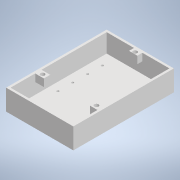
# Autodesk Inventor part: корпус
Saved by Autodesk Inventor 2022 (Build 260153000, 153)
## iProperties
Created: 2022-10-20
Part Number: корпус
Material: Типовые
Document SubType Name: Modeling
Designer: Robo0
Density: 1 g/cm^3
Appearance: По умолчанию
Author: Robo0
Autodesk Inventor part; units mm, degrees
ref_plane "YZ Plane" through (0, 0, 0) normal (1, 0, 0) x (0, 1, 0)
ref_plane "XZ Plane" through (0, 0, 0) normal (0, 1, 0) x (-1, 0, 0)
ref_plane "XY Plane" through (0, 0, 0) normal (0, 0, 1) x (1, 0, 0)
sketch "Эскиз1" plane through (0, 0, 0) normal (0, 1, 0) x (-1, 0, 0)
  line L0 (0, 0) -> (200, 0)
  line L1 (200, 0) -> (200, 200)
  line L2 (200, 200) -> (0, 200)
  line L3 (0, 200) -> (0, 0)
  dimension "d0" = 200
  dimension "d1" = 200
  constraints: 8 end point, 2 parallel, 1 horizontal, 1 perpendicular
  measures "d0" distance of L2.end L1.end
  measures "d1" distance of L1.end L0.end
extrude "Выдавливание1" add sketch "Эскиз1" along normal blind 3
sketch "Эскиз2" plane through (0, 3, 0) normal (0, 1, 0) x (1, 0, 0)
  line L0 (-200, 0) -> (-200, -200) projected
  line L1 (-200, -200) -> (0, -200) projected
  line L2 (0, -200) -> (0, 0) projected
  line L3 (0, 0) -> (-200, 0) projected
  line L4 (0, -200) -> (0, 0) projected
  line L5 (0, 0) -> (-90.778, 0)
  line L6 (-90.778, 0) -> (-90.778, -135.834)
  line L7 (-90.778, -135.834) -> (0, -135.834)
  line L8 (0, -135.834) -> (0, 0)
  constraints: 8 end point, 2 parallel, 1 horizontal, 1 perpendicular
extrude "Выдавливание2" cut sketch "Эскиз2" against normal blind 3 contours L3 L6 L7 L2 L1 L0
sketch "Эскиз3" plane through (0, 3, 0) normal (0, 1, 0) x (1, 0, 0)
  line L0 (-90.778, 0) -> (-90.778, -135.834) projected
  line L1 (-90.778, -135.834) -> (0, -135.834) projected
  line L2 (0, -135.834) -> (0, 0) projected
  line L3 (0, 0) -> (-90.778, 0) projected
  line L4 (-87.778, -132.834) -> (-3, -132.834)
  line L5 (-3, -132.834) -> (-3, -3)
  line L6 (-3, -3) -> (-87.778, -3)
  line L7 (-87.778, -3) -> (-87.778, -132.834)
  dimension "d6" = 3
  dimension "d7" = 3
  dimension "d8" = 3
  dimension "d9" = 3
  constraints: 8 end point, 2 parallel, 1 horizontal, 1 perpendicular
  measures "d6" distance between parallel lines of L0 L7
  measures "d7" distance between parallel lines of L6 L3
  measures "d8" distance between parallel lines of L2 L5
  measures "d9" distance between parallel lines of L1 L4
extrude "Выдавливание3" add sketch "Эскиз3" along normal blind 25
sketch "Эскиз4" plane through (0, 28, 0) normal (0, 1, 0) x (1, 0, 0)
  line L0 (-87.778, -3) -> (-3, -3) projected
  line L1 (-87.778, -132.834) -> (-87.778, -3) projected
  line L2 (-3, -3) -> (-3, -132.834) projected
  circle A0 centre (-81.778, -95.6228) radius 2.75
  circle A1 centre (-9, -95.6228) radius 2.75
  circle A2 centre (-45.389, -7) radius 2.75
  line L3 (-87.778, -99.5857) -> (-76.0264, -99.5857)
  line L4 (-76.0264, -99.5857) -> (-76.0264, -91)
  line L5 (-76.0264, -91) -> (-87.778, -91)
  line L6 (-87.778, -91) -> (-87.778, -99.5857)
  line L7 (-50.872, -3) -> (-39.6049, -3)
  line L8 (-39.6049, -3) -> (-39.6049, -9.75)
  line L9 (-39.6049, -9.75) -> (-50.872, -9.75)
  line L10 (-50.872, -9.75) -> (-50.872, -3)
  line L11 (-3, -91) -> (-13.2714, -91)
  line L12 (-13.2714, -91) -> (-13.2714, -100.2408)
  line L13 (-13.2714, -100.2408) -> (-3, -100.2408)
  line L14 (-3, -100.2408) -> (-3, -91)
  line L15 (-36, -90) -> (-62, -90) projected
  point P0 (0, 0)
  point P1 (-45.389, -9.75)
  point P2 (-3, -100.2408)
  dimension "d12" = 5.5
  dimension "d13" = 6
  dimension "d14" = 5.5
  dimension "d15" = 6
  dimension "d16" = 5.5
  dimension "d17" = 4
  dimension "d18" = 1
  dimension "d19" = 4.6227
  constraints: 24 end point, 6 parallel, 4 point on line, 3 centre point, 3 horizontal, 3 perpendicular
  measures "d12" diameter of A0
  measures "d13" distance from line of A0.centre L1
  measures "d14" diameter of A1
  measures "d15" distance from line of A1.centre L2
  measures "d16" diameter of A2
  measures "d17" distance from line of A2.centre L0
  measures "d18" distance between parallel lines of L5 L15
  measures "d19" distance from line of L5 A0.centre
extrude "Выдавливание4" add sketch "Эскиз4" against normal blind 10
sketch "Эскиз5" plane through (-90.778, 0, 0) normal (-1, 0, 0) x (0, 0, 1)
  point P0 (0, 0)
sketch "Эскиз6" plane through (-90.778, 0, 0) normal (-1, 0, 0) x (0, 0, 1)
  line L0 (123, 6.5) -> (123, 0.5) projected
  line L1 (129, 6.5) -> (123, 6.5) projected
  line L2 (129, 0.5) -> (129, 6.5) projected
  line L3 (129.6397, 6.975) -> (122.4748, 6.975)
  line L4 (122.4748, 6.975) -> (122.4748, 0.5)
  line L5 (122.4748, 0.5) -> (129.6397, 0.5)
  line L6 (129.6397, 0.5) -> (129.6397, 6.975)
  point P0 (0, 0)
  constraints: 8 end point, 2 parallel, 1 horizontal, 1 perpendicular
extrude "Выдавливание5" cut sketch "Эскиз6" against normal blind 10
sketch "Эскиз7" plane through (0, 0, 0) normal (0, -1, 0) x (1, 0, 0)
  spline S0 degree 3 poles (-76.75, 18.5) (-76.7941, 18.5) (-76.8383, 18.5019) (-76.8822, 18.5058) (-76.939, 18.5109) (-76.9955, 18.5191) (-77.0514, 18.5306) (-77.1245, 18.5456) (-77.1965, 18.566) (-77.2665, 18.5917) (-77.3391, 18.6184) (-77.4096, 18.6506) (-77.4772, 18.688) (-77.5359, 18.7206) (-77.5924, 18.7571) (-77.6462, 18.7972) (-77.688, 18.8283) (-77.7282, 18.8617) (-77.7666, 18.897) (-77.8049, 18.9323) (-77.8413, 18.9696) (-77.8758, 19.0087) (-77.9079, 19.0452) (-77.9382, 19.0832) (-77.9666, 19.1226) (-77.993, 19.1592) (-78.0178, 19.1971) (-78.0408, 19.2359) (-78.0657, 19.278) (-78.0886, 19.3213) (-78.1092, 19.3656) (-78.1329, 19.4162) (-78.1537, 19.4682) (-78.1715, 19.5212) (-78.1907, 19.578) (-78.2064, 19.636) (-78.2186, 19.6948) (-78.2287, 19.7432) (-78.2363, 19.7921) (-78.2416, 19.8412) (-78.2457, 19.88) (-78.2483, 19.9189) (-78.2494, 19.9579) (-78.2498, 19.9719) (-78.25, 19.986) (-78.25, 20) (-78.25, 20.0174) (-78.2497, 20.0348) (-78.2491, 20.0521) (-78.248, 20.0835) (-78.2459, 20.1149) (-78.2429, 20.1461) (-78.2385, 20.1907) (-78.2321, 20.2351) (-78.2238, 20.2791) (-78.2135, 20.3334) (-78.2003, 20.3871) (-78.1841, 20.4399) (-78.1648, 20.5026) (-78.1414, 20.5641) (-78.1141, 20.6238) (-78.091, 20.6745) (-78.065, 20.7238) (-78.0363, 20.7716) (-78.0113, 20.8134) (-77.9842, 20.8539) (-77.9552, 20.893) (-77.9283, 20.9293) (-77.8998, 20.9643) (-77.8698, 20.998) (-77.8375, 21.0343) (-77.8034, 21.0689) (-77.7678, 21.1019) (-77.727, 21.1395) (-77.6843, 21.1748) (-77.6396, 21.2077) (-77.5923, 21.2426) (-77.5428, 21.2747) (-77.4916, 21.3038) (-77.4405, 21.3329) (-77.3877, 21.359) (-77.3335, 21.3818) (-77.2826, 21.4034) (-77.2304, 21.4221) (-77.1774, 21.4378) (-77.131, 21.4516) (-77.084, 21.4631) (-77.0365, 21.4724) (-76.9925, 21.4809) (-76.9481, 21.4875) (-76.9034, 21.4921) (-76.8622, 21.4964) (-76.8209, 21.4989) (-76.7795, 21.4997) (-76.7696, 21.4999) (-76.7598, 21.5) (-76.75, 21.5) (-76.7184, 21.5) (-76.6869, 21.499) (-76.6554, 21.497) (-76.6107, 21.4942) (-76.5661, 21.4894) (-76.5218, 21.4825) (-76.4741, 21.4752) (-76.4268, 21.4656) (-76.3801, 21.4537) (-76.3266, 21.4401) (-76.274, 21.4235) (-76.2224, 21.4042) (-76.1676, 21.3836) (-76.1141, 21.3598) (-76.0621, 21.333) (-76.0101, 21.3061) (-75.9596, 21.2762) (-75.911, 21.2434) (-75.8652, 21.2125) (-75.8211, 21.1791) (-75.779, 21.1433) (-75.7262, 21.0985) (-75.6765, 21.0499) (-75.6303, 20.9982) (-75.5771, 20.9384) (-75.5286, 20.8744) (-75.4855, 20.8069) (-75.4443, 20.7423) (-75.408, 20.6745) (-75.3771, 20.6042) (-75.3546, 20.5531) (-75.3349, 20.5007) (-75.3182, 20.4473) (-75.3042, 20.4024) (-75.2923, 20.3568) (-75.2826, 20.3108) (-75.2735, 20.2682) (-75.2664, 20.2251) (-75.2611, 20.1819) (-75.2562, 20.1421) (-75.2529, 20.1021) (-75.2513, 20.062) (-75.2504, 20.0413) (-75.25, 20.0207) (-75.25, 20) (-75.25, 19.9892) (-75.2501, 19.9785) (-75.2503, 19.9677) (-75.251, 19.9363) (-75.2527, 19.9049) (-75.2553, 19.8736) (-75.259, 19.8301) (-75.2646, 19.7868) (-75.2721, 19.7437) (-75.2813, 19.6904) (-75.2934, 19.6375) (-75.3084, 19.5855) (-75.3262, 19.5235) (-75.3481, 19.4626) (-75.3738, 19.4034) (-75.3959, 19.3522) (-75.4209, 19.3023) (-75.4487, 19.254) (-75.4729, 19.2117) (-75.4992, 19.1707) (-75.5274, 19.131) (-75.5535, 19.0942) (-75.5813, 19.0586) (-75.6107, 19.0243) (-75.6423, 18.9874) (-75.6757, 18.9521) (-75.7107, 18.9184) (-75.7507, 18.88) (-75.7928, 18.8438) (-75.8367, 18.8101) (-75.8834, 18.7742) (-75.9322, 18.7411) (-75.9828, 18.711) (-76.0343, 18.6804) (-76.0876, 18.6529) (-76.1424, 18.6286) (-76.1949, 18.6053) (-76.2489, 18.585) (-76.3038, 18.5679) (-76.3541, 18.5522) (-76.4053, 18.5392) (-76.457, 18.5289) (-76.5064, 18.5191) (-76.5563, 18.5117) (-76.6064, 18.5069) (-76.6541, 18.5023) (-76.702, 18.5) (-76.75, 18.5) knots 0 0 0 0 0.014027 0.014027 0.014027 0.032151 0.032151 0.032151 0.055886 0.055886 0.055886 0.080494 0.080494 0.080494 0.10188 0.10188 0.10188 0.118509 0.118509 0.118509 0.135113 0.135113 0.135113 0.150598 0.150598 0.150598 0.164992 0.164992 0.164992 0.180561 0.180561 0.180561 0.198348 0.198348 0.198348 0.217433 0.217433 0.217433 0.23315 0.23315 0.23315 0.245536 0.245536 0.245536 0.249999 0.249999 0.249999 0.255524 0.255524 0.255524 0.265505 0.265505 0.265505 0.27974 0.27974 0.27974 0.297306 0.297306 0.297306 0.318194 0.318194 0.318194 0.335939 0.335939 0.335939 0.351456 0.351456 0.351456 0.36584 0.36584 0.36584 0.381321 0.381321 0.381321 0.398988 0.398988 0.398988 0.417741 0.417741 0.417741 0.436466 0.436466 0.436466 0.454074 0.454074 0.454074 0.469453 0.469453 0.469453 0.483718 0.483718 0.483718 0.496876 0.496876 0.496876 0.499998 0.499998 0.499998 0.51003 0.51003 0.51003 0.524271 0.524271 0.524271 0.539608 0.539608 0.539608 0.557137 0.557137 0.557137 0.575761 0.575761 0.575761 0.594424 0.594424 0.594424 0.612031 0.612031 0.612031 0.634137 0.634137 0.634137 0.659646 0.659646 0.659646 0.684077 0.684077 0.684077 0.701865 0.701865 0.701865 0.716826 0.716826 0.716826 0.730685 0.730685 0.730685 0.743429 0.743429 0.743429 0.749997 0.749997 0.749997 0.753416 0.753416 0.753416 0.763398 0.763398 0.763398 0.777282 0.777282 0.777282 0.794497 0.794497 0.794497 0.815037 0.815037 0.815037 0.832783 0.832783 0.832783 0.848301 0.848301 0.848301 0.862688 0.862688 0.862688 0.878174 0.878174 0.878174 0.895845 0.895845 0.895845 0.914604 0.914604 0.914604 0.933679 0.933679 0.933679 0.951984 0.951984 0.951984 0.968755 0.968755 0.968755 0.984759 0.984759 0.984759 1 1 1 1 projected
  spline S1 degree 3 poles (-76.75, 38.5) (-76.7941, 38.5) (-76.8383, 38.5019) (-76.8822, 38.5058) (-76.939, 38.5109) (-76.9955, 38.5191) (-77.0514, 38.5306) (-77.1245, 38.5456) (-77.1965, 38.566) (-77.2665, 38.5917) (-77.3391, 38.6184) (-77.4096, 38.6506) (-77.4772, 38.688) (-77.5359, 38.7206) (-77.5924, 38.7571) (-77.6462, 38.7972) (-77.688, 38.8283) (-77.7282, 38.8617) (-77.7666, 38.897) (-77.8049, 38.9323) (-77.8413, 38.9696) (-77.8758, 39.0087) (-77.9079, 39.0452) (-77.9382, 39.0832) (-77.9666, 39.1226) (-77.993, 39.1592) (-78.0178, 39.1971) (-78.0408, 39.2359) (-78.0657, 39.278) (-78.0886, 39.3213) (-78.1092, 39.3656) (-78.1329, 39.4162) (-78.1537, 39.4682) (-78.1715, 39.5212) (-78.1907, 39.578) (-78.2064, 39.636) (-78.2186, 39.6948) (-78.2287, 39.7432) (-78.2363, 39.7921) (-78.2416, 39.8412) (-78.2457, 39.88) (-78.2483, 39.9189) (-78.2494, 39.9579) (-78.2498, 39.9719) (-78.25, 39.986) (-78.25, 40) (-78.25, 40.0174) (-78.2497, 40.0348) (-78.2491, 40.0521) (-78.248, 40.0835) (-78.2459, 40.1149) (-78.2429, 40.1461) (-78.2385, 40.1907) (-78.2321, 40.2351) (-78.2238, 40.2791) (-78.2135, 40.3334) (-78.2003, 40.3871) (-78.1841, 40.4399) (-78.1648, 40.5026) (-78.1414, 40.5641) (-78.1141, 40.6238) (-78.091, 40.6745) (-78.065, 40.7238) (-78.0363, 40.7716) (-78.0113, 40.8134) (-77.9842, 40.8539) (-77.9552, 40.893) (-77.9283, 40.9293) (-77.8998, 40.9643) (-77.8698, 40.998) (-77.8375, 41.0343) (-77.8034, 41.0689) (-77.7678, 41.1019) (-77.727, 41.1395) (-77.6843, 41.1748) (-77.6396, 41.2077) (-77.5923, 41.2426) (-77.5428, 41.2747) (-77.4916, 41.3038) (-77.4405, 41.3329) (-77.3877, 41.359) (-77.3335, 41.3818) (-77.2826, 41.4034) (-77.2304, 41.4221) (-77.1774, 41.4378) (-77.131, 41.4516) (-77.084, 41.4631) (-77.0365, 41.4724) (-76.9925, 41.4809) (-76.9481, 41.4875) (-76.9034, 41.4921) (-76.8622, 41.4964) (-76.8209, 41.4989) (-76.7795, 41.4997) (-76.7696, 41.4999) (-76.7598, 41.5) (-76.75, 41.5) (-76.7184, 41.5) (-76.6869, 41.499) (-76.6554, 41.497) (-76.6107, 41.4942) (-76.5661, 41.4894) (-76.5218, 41.4825) (-76.4741, 41.4752) (-76.4268, 41.4656) (-76.3801, 41.4537) (-76.3266, 41.4401) (-76.274, 41.4235) (-76.2224, 41.4042) (-76.1676, 41.3836) (-76.1141, 41.3598) (-76.0621, 41.333) (-76.0101, 41.3061) (-75.9596, 41.2762) (-75.911, 41.2434) (-75.8652, 41.2125) (-75.8211, 41.1791) (-75.779, 41.1433) (-75.7262, 41.0985) (-75.6765, 41.0499) (-75.6303, 40.9982) (-75.5771, 40.9384) (-75.5286, 40.8744) (-75.4855, 40.8069) (-75.4443, 40.7423) (-75.408, 40.6745) (-75.3771, 40.6042) (-75.3546, 40.5531) (-75.3349, 40.5007) (-75.3182, 40.4473) (-75.3042, 40.4024) (-75.2923, 40.3568) (-75.2826, 40.3108) (-75.2735, 40.2682) (-75.2664, 40.2251) (-75.2611, 40.1819) (-75.2562, 40.1421) (-75.2529, 40.1021) (-75.2513, 40.062) (-75.2504, 40.0413) (-75.25, 40.0207) (-75.25, 40) (-75.25, 39.9892) (-75.2501, 39.9785) (-75.2503, 39.9677) (-75.251, 39.9363) (-75.2527, 39.9049) (-75.2553, 39.8736) (-75.259, 39.8301) (-75.2646, 39.7868) (-75.2721, 39.7437) (-75.2813, 39.6904) (-75.2934, 39.6375) (-75.3084, 39.5855) (-75.3262, 39.5235) (-75.3481, 39.4626) (-75.3738, 39.4034) (-75.3959, 39.3522) (-75.4209, 39.3023) (-75.4487, 39.254) (-75.4729, 39.2117) (-75.4992, 39.1707) (-75.5274, 39.131) (-75.5535, 39.0942) (-75.5813, 39.0586) (-75.6107, 39.0243) (-75.6423, 38.9874) (-75.6757, 38.9521) (-75.7107, 38.9184) (-75.7507, 38.88) (-75.7928, 38.8438) (-75.8367, 38.8101) (-75.8834, 38.7742) (-75.9322, 38.7411) (-75.9828, 38.711) (-76.0343, 38.6804) (-76.0876, 38.6529) (-76.1424, 38.6286) (-76.1949, 38.6053) (-76.2489, 38.585) (-76.3038, 38.5679) (-76.3541, 38.5522) (-76.4053, 38.5392) (-76.457, 38.5289) (-76.5064, 38.5191) (-76.5563, 38.5117) (-76.6064, 38.5069) (-76.6541, 38.5023) (-76.702, 38.5) (-76.75, 38.5) knots 0 0 0 0 0.014027 0.014027 0.014027 0.032151 0.032151 0.032151 0.055886 0.055886 0.055886 0.080494 0.080494 0.080494 0.10188 0.10188 0.10188 0.118509 0.118509 0.118509 0.135113 0.135113 0.135113 0.150598 0.150598 0.150598 0.164992 0.164992 0.164992 0.180561 0.180561 0.180561 0.198348 0.198348 0.198348 0.217433 0.217433 0.217433 0.23315 0.23315 0.23315 0.245536 0.245536 0.245536 0.249999 0.249999 0.249999 0.255524 0.255524 0.255524 0.265505 0.265505 0.265505 0.27974 0.27974 0.27974 0.297306 0.297306 0.297306 0.318194 0.318194 0.318194 0.335939 0.335939 0.335939 0.351456 0.351456 0.351456 0.36584 0.36584 0.36584 0.381321 0.381321 0.381321 0.398988 0.398988 0.398988 0.417741 0.417741 0.417741 0.436466 0.436466 0.436466 0.454074 0.454074 0.454074 0.469453 0.469453 0.469453 0.483718 0.483718 0.483718 0.496876 0.496876 0.496876 0.499998 0.499998 0.499998 0.51003 0.51003 0.51003 0.524271 0.524271 0.524271 0.539608 0.539608 0.539608 0.557137 0.557137 0.557137 0.575761 0.575761 0.575761 0.594424 0.594424 0.594424 0.612031 0.612031 0.612031 0.634137 0.634137 0.634137 0.659646 0.659646 0.659646 0.684077 0.684077 0.684077 0.701865 0.701865 0.701865 0.716826 0.716826 0.716826 0.730685 0.730685 0.730685 0.743429 0.743429 0.743429 0.749997 0.749997 0.749997 0.753416 0.753416 0.753416 0.763398 0.763398 0.763398 0.777282 0.777282 0.777282 0.794497 0.794497 0.794497 0.815037 0.815037 0.815037 0.832783 0.832783 0.832783 0.848301 0.848301 0.848301 0.862688 0.862688 0.862688 0.878174 0.878174 0.878174 0.895845 0.895845 0.895845 0.914604 0.914604 0.914604 0.933679 0.933679 0.933679 0.951984 0.951984 0.951984 0.968755 0.968755 0.968755 0.984759 0.984759 0.984759 1 1 1 1 projected
  spline S2 degree 3 poles (-76.75, 58.5) (-76.7941, 58.5) (-76.8383, 58.5019) (-76.8822, 58.5058) (-76.939, 58.5109) (-76.9955, 58.5191) (-77.0514, 58.5306) (-77.1245, 58.5456) (-77.1965, 58.566) (-77.2665, 58.5917) (-77.3391, 58.6184) (-77.4096, 58.6506) (-77.4772, 58.688) (-77.5359, 58.7206) (-77.5924, 58.7571) (-77.6462, 58.7972) (-77.688, 58.8283) (-77.7282, 58.8617) (-77.7666, 58.897) (-77.8049, 58.9323) (-77.8413, 58.9696) (-77.8758, 59.0087) (-77.9079, 59.0452) (-77.9382, 59.0832) (-77.9666, 59.1226) (-77.993, 59.1592) (-78.0178, 59.1971) (-78.0408, 59.2359) (-78.0657, 59.278) (-78.0886, 59.3213) (-78.1092, 59.3656) (-78.1329, 59.4162) (-78.1537, 59.4682) (-78.1715, 59.5212) (-78.1907, 59.578) (-78.2064, 59.636) (-78.2186, 59.6948) (-78.2287, 59.7432) (-78.2363, 59.7921) (-78.2416, 59.8412) (-78.2457, 59.88) (-78.2483, 59.9189) (-78.2494, 59.9579) (-78.2498, 59.9719) (-78.25, 59.986) (-78.25, 60) (-78.25, 60.0174) (-78.2497, 60.0348) (-78.2491, 60.0521) (-78.248, 60.0835) (-78.2459, 60.1149) (-78.2429, 60.1461) (-78.2385, 60.1907) (-78.2321, 60.2351) (-78.2238, 60.2791) (-78.2135, 60.3334) (-78.2003, 60.3871) (-78.1841, 60.4399) (-78.1648, 60.5026) (-78.1414, 60.5641) (-78.1141, 60.6238) (-78.091, 60.6745) (-78.065, 60.7238) (-78.0363, 60.7716) (-78.0113, 60.8134) (-77.9842, 60.8539) (-77.9552, 60.893) (-77.9283, 60.9293) (-77.8998, 60.9643) (-77.8698, 60.998) (-77.8375, 61.0343) (-77.8034, 61.0689) (-77.7678, 61.1019) (-77.727, 61.1395) (-77.6843, 61.1748) (-77.6396, 61.2077) (-77.5923, 61.2426) (-77.5428, 61.2747) (-77.4916, 61.3038) (-77.4405, 61.3329) (-77.3877, 61.359) (-77.3335, 61.3818) (-77.2826, 61.4034) (-77.2304, 61.4221) (-77.1774, 61.4378) (-77.131, 61.4516) (-77.084, 61.4631) (-77.0365, 61.4724) (-76.9925, 61.4809) (-76.9481, 61.4875) (-76.9034, 61.4921) (-76.8622, 61.4964) (-76.8209, 61.4989) (-76.7795, 61.4997) (-76.7696, 61.4999) (-76.7598, 61.5) (-76.75, 61.5) (-76.7184, 61.5) (-76.6869, 61.499) (-76.6554, 61.497) (-76.6107, 61.4942) (-76.5661, 61.4894) (-76.5218, 61.4825) (-76.4741, 61.4752) (-76.4268, 61.4656) (-76.3801, 61.4537) (-76.3266, 61.4401) (-76.274, 61.4235) (-76.2224, 61.4042) (-76.1676, 61.3836) (-76.1141, 61.3598) (-76.0621, 61.333) (-76.0101, 61.3061) (-75.9596, 61.2762) (-75.911, 61.2434) (-75.8652, 61.2125) (-75.8211, 61.1791) (-75.779, 61.1433) (-75.7262, 61.0985) (-75.6765, 61.0499) (-75.6303, 60.9982) (-75.5771, 60.9384) (-75.5286, 60.8744) (-75.4855, 60.8069) (-75.4443, 60.7423) (-75.408, 60.6745) (-75.3771, 60.6042) (-75.3546, 60.5531) (-75.3349, 60.5007) (-75.3182, 60.4473) (-75.3042, 60.4024) (-75.2923, 60.3568) (-75.2826, 60.3108) (-75.2735, 60.2682) (-75.2664, 60.2251) (-75.2611, 60.1819) (-75.2562, 60.1421) (-75.2529, 60.1021) (-75.2513, 60.062) (-75.2504, 60.0413) (-75.25, 60.0207) (-75.25, 60) (-75.25, 59.9892) (-75.2501, 59.9785) (-75.2503, 59.9677) (-75.251, 59.9363) (-75.2527, 59.9049) (-75.2553, 59.8736) (-75.259, 59.8301) (-75.2646, 59.7868) (-75.2721, 59.7437) (-75.2813, 59.6904) (-75.2934, 59.6375) (-75.3084, 59.5855) (-75.3262, 59.5235) (-75.3481, 59.4626) (-75.3738, 59.4034) (-75.3959, 59.3522) (-75.4209, 59.3023) (-75.4487, 59.254) (-75.4729, 59.2117) (-75.4992, 59.1707) (-75.5274, 59.131) (-75.5535, 59.0942) (-75.5813, 59.0586) (-75.6107, 59.0243) (-75.6423, 58.9874) (-75.6757, 58.9521) (-75.7107, 58.9184) (-75.7507, 58.88) (-75.7928, 58.8438) (-75.8367, 58.8101) (-75.8834, 58.7742) (-75.9322, 58.7411) (-75.9828, 58.711) (-76.0343, 58.6804) (-76.0876, 58.6529) (-76.1424, 58.6286) (-76.1949, 58.6053) (-76.2489, 58.585) (-76.3038, 58.5679) (-76.3541, 58.5522) (-76.4053, 58.5392) (-76.457, 58.5289) (-76.5064, 58.5191) (-76.5563, 58.5117) (-76.6064, 58.5069) (-76.6541, 58.5023) (-76.702, 58.5) (-76.75, 58.5) knots 0 0 0 0 0.014027 0.014027 0.014027 0.032151 0.032151 0.032151 0.055886 0.055886 0.055886 0.080494 0.080494 0.080494 0.10188 0.10188 0.10188 0.118509 0.118509 0.118509 0.135113 0.135113 0.135113 0.150598 0.150598 0.150598 0.164992 0.164992 0.164992 0.180561 0.180561 0.180561 0.198348 0.198348 0.198348 0.217433 0.217433 0.217433 0.23315 0.23315 0.23315 0.245536 0.245536 0.245536 0.249999 0.249999 0.249999 0.255524 0.255524 0.255524 0.265505 0.265505 0.265505 0.27974 0.27974 0.27974 0.297306 0.297306 0.297306 0.318194 0.318194 0.318194 0.335939 0.335939 0.335939 0.351456 0.351456 0.351456 0.36584 0.36584 0.36584 0.381321 0.381321 0.381321 0.398988 0.398988 0.398988 0.417741 0.417741 0.417741 0.436466 0.436466 0.436466 0.454074 0.454074 0.454074 0.469453 0.469453 0.469453 0.483718 0.483718 0.483718 0.496876 0.496876 0.496876 0.499998 0.499998 0.499998 0.51003 0.51003 0.51003 0.524271 0.524271 0.524271 0.539608 0.539608 0.539608 0.557137 0.557137 0.557137 0.575761 0.575761 0.575761 0.594424 0.594424 0.594424 0.612031 0.612031 0.612031 0.634137 0.634137 0.634137 0.659646 0.659646 0.659646 0.684077 0.684077 0.684077 0.701865 0.701865 0.701865 0.716826 0.716826 0.716826 0.730685 0.730685 0.730685 0.743429 0.743429 0.743429 0.749997 0.749997 0.749997 0.753416 0.753416 0.753416 0.763398 0.763398 0.763398 0.777282 0.777282 0.777282 0.794497 0.794497 0.794497 0.815037 0.815037 0.815037 0.832783 0.832783 0.832783 0.848301 0.848301 0.848301 0.862688 0.862688 0.862688 0.878174 0.878174 0.878174 0.895845 0.895845 0.895845 0.914604 0.914604 0.914604 0.933679 0.933679 0.933679 0.951984 0.951984 0.951984 0.968755 0.968755 0.968755 0.984759 0.984759 0.984759 1 1 1 1 projected
  spline S3 degree 3 poles (-76.75, 78.5) (-76.7941, 78.5) (-76.8383, 78.5019) (-76.8822, 78.5058) (-76.939, 78.5109) (-76.9955, 78.5191) (-77.0514, 78.5306) (-77.1245, 78.5456) (-77.1965, 78.566) (-77.2665, 78.5917) (-77.3391, 78.6184) (-77.4096, 78.6506) (-77.4772, 78.688) (-77.5359, 78.7206) (-77.5924, 78.7571) (-77.6462, 78.7972) (-77.688, 78.8283) (-77.7282, 78.8617) (-77.7666, 78.897) (-77.8049, 78.9323) (-77.8413, 78.9696) (-77.8758, 79.0087) (-77.9079, 79.0452) (-77.9382, 79.0832) (-77.9666, 79.1226) (-77.993, 79.1592) (-78.0178, 79.1971) (-78.0408, 79.2359) (-78.0657, 79.278) (-78.0886, 79.3213) (-78.1092, 79.3656) (-78.1329, 79.4162) (-78.1537, 79.4682) (-78.1715, 79.5212) (-78.1907, 79.578) (-78.2064, 79.636) (-78.2186, 79.6948) (-78.2287, 79.7432) (-78.2363, 79.7921) (-78.2416, 79.8412) (-78.2457, 79.88) (-78.2483, 79.9189) (-78.2494, 79.9579) (-78.2498, 79.9719) (-78.25, 79.986) (-78.25, 80) (-78.25, 80.0174) (-78.2497, 80.0348) (-78.2491, 80.0521) (-78.248, 80.0835) (-78.2459, 80.1149) (-78.2429, 80.1461) (-78.2385, 80.1907) (-78.2321, 80.2351) (-78.2238, 80.2791) (-78.2135, 80.3334) (-78.2003, 80.3871) (-78.1841, 80.4399) (-78.1648, 80.5026) (-78.1414, 80.5641) (-78.1141, 80.6238) (-78.091, 80.6745) (-78.065, 80.7238) (-78.0363, 80.7716) (-78.0113, 80.8134) (-77.9842, 80.8539) (-77.9552, 80.893) (-77.9283, 80.9293) (-77.8998, 80.9643) (-77.8698, 80.998) (-77.8375, 81.0343) (-77.8034, 81.0689) (-77.7678, 81.1019) (-77.727, 81.1395) (-77.6843, 81.1748) (-77.6396, 81.2077) (-77.5923, 81.2426) (-77.5428, 81.2747) (-77.4916, 81.3038) (-77.4405, 81.3329) (-77.3877, 81.359) (-77.3335, 81.3818) (-77.2826, 81.4034) (-77.2304, 81.4221) (-77.1774, 81.4378) (-77.131, 81.4516) (-77.084, 81.4631) (-77.0365, 81.4724) (-76.9925, 81.4809) (-76.9481, 81.4875) (-76.9034, 81.4921) (-76.8622, 81.4964) (-76.8209, 81.4989) (-76.7795, 81.4997) (-76.7696, 81.4999) (-76.7598, 81.5) (-76.75, 81.5) (-76.7184, 81.5) (-76.6869, 81.499) (-76.6554, 81.497) (-76.6107, 81.4942) (-76.5661, 81.4894) (-76.5218, 81.4825) (-76.4741, 81.4752) (-76.4268, 81.4656) (-76.3801, 81.4537) (-76.3266, 81.4401) (-76.274, 81.4235) (-76.2224, 81.4042) (-76.1676, 81.3836) (-76.1141, 81.3598) (-76.0621, 81.333) (-76.0101, 81.3061) (-75.9596, 81.2762) (-75.911, 81.2434) (-75.8652, 81.2125) (-75.8211, 81.1791) (-75.779, 81.1433) (-75.7262, 81.0985) (-75.6765, 81.0499) (-75.6303, 80.9982) (-75.5771, 80.9384) (-75.5286, 80.8744) (-75.4855, 80.8069) (-75.4443, 80.7423) (-75.408, 80.6745) (-75.3771, 80.6042) (-75.3546, 80.5531) (-75.3349, 80.5007) (-75.3182, 80.4473) (-75.3042, 80.4024) (-75.2923, 80.3568) (-75.2826, 80.3108) (-75.2735, 80.2682) (-75.2664, 80.2251) (-75.2611, 80.1819) (-75.2562, 80.1421) (-75.2529, 80.1021) (-75.2513, 80.062) (-75.2504, 80.0413) (-75.25, 80.0207) (-75.25, 80) (-75.25, 79.9892) (-75.2501, 79.9785) (-75.2503, 79.9677) (-75.251, 79.9363) (-75.2527, 79.9049) (-75.2553, 79.8736) (-75.259, 79.8301) (-75.2646, 79.7868) (-75.2721, 79.7437) (-75.2813, 79.6904) (-75.2934, 79.6375) (-75.3084, 79.5855) (-75.3262, 79.5235) (-75.3481, 79.4626) (-75.3738, 79.4034) (-75.3959, 79.3522) (-75.4209, 79.3023) (-75.4487, 79.254) (-75.4729, 79.2117) (-75.4992, 79.1707) (-75.5274, 79.131) (-75.5535, 79.0942) (-75.5813, 79.0586) (-75.6107, 79.0243) (-75.6423, 78.9874) (-75.6757, 78.9521) (-75.7107, 78.9184) (-75.7507, 78.88) (-75.7928, 78.8438) (-75.8367, 78.8101) (-75.8834, 78.7742) (-75.9322, 78.7411) (-75.9828, 78.711) (-76.0343, 78.6804) (-76.0876, 78.6529) (-76.1424, 78.6286) (-76.1949, 78.6053) (-76.2489, 78.585) (-76.3038, 78.5679) (-76.3541, 78.5522) (-76.4053, 78.5392) (-76.457, 78.5289) (-76.5064, 78.5191) (-76.5563, 78.5117) (-76.6064, 78.5069) (-76.6541, 78.5023) (-76.702, 78.5) (-76.75, 78.5) knots 0 0 0 0 0.014027 0.014027 0.014027 0.032151 0.032151 0.032151 0.055886 0.055886 0.055886 0.080494 0.080494 0.080494 0.10188 0.10188 0.10188 0.118509 0.118509 0.118509 0.135113 0.135113 0.135113 0.150598 0.150598 0.150598 0.164992 0.164992 0.164992 0.180561 0.180561 0.180561 0.198348 0.198348 0.198348 0.217433 0.217433 0.217433 0.23315 0.23315 0.23315 0.245536 0.245536 0.245536 0.249999 0.249999 0.249999 0.255524 0.255524 0.255524 0.265505 0.265505 0.265505 0.27974 0.27974 0.27974 0.297306 0.297306 0.297306 0.318194 0.318194 0.318194 0.335939 0.335939 0.335939 0.351456 0.351456 0.351456 0.36584 0.36584 0.36584 0.381321 0.381321 0.381321 0.398988 0.398988 0.398988 0.417741 0.417741 0.417741 0.436466 0.436466 0.436466 0.454074 0.454074 0.454074 0.469453 0.469453 0.469453 0.483718 0.483718 0.483718 0.496876 0.496876 0.496876 0.499998 0.499998 0.499998 0.51003 0.51003 0.51003 0.524271 0.524271 0.524271 0.539608 0.539608 0.539608 0.557137 0.557137 0.557137 0.575761 0.575761 0.575761 0.594424 0.594424 0.594424 0.612031 0.612031 0.612031 0.634137 0.634137 0.634137 0.659646 0.659646 0.659646 0.684077 0.684077 0.684077 0.701865 0.701865 0.701865 0.716826 0.716826 0.716826 0.730685 0.730685 0.730685 0.743429 0.743429 0.743429 0.749997 0.749997 0.749997 0.753416 0.753416 0.753416 0.763398 0.763398 0.763398 0.777282 0.777282 0.777282 0.794497 0.794497 0.794497 0.815037 0.815037 0.815037 0.832783 0.832783 0.832783 0.848301 0.848301 0.848301 0.862688 0.862688 0.862688 0.878174 0.878174 0.878174 0.895845 0.895845 0.895845 0.914604 0.914604 0.914604 0.933679 0.933679 0.933679 0.951984 0.951984 0.951984 0.968755 0.968755 0.968755 0.984759 0.984759 0.984759 1 1 1 1 projected
  spline S4 degree 3 poles (-21.25, 58.5) (-21.2941, 58.5) (-21.3383, 58.5019) (-21.3822, 58.5058) (-21.439, 58.5109) (-21.4955, 58.5191) (-21.5514, 58.5306) (-21.6245, 58.5456) (-21.6965, 58.566) (-21.7665, 58.5917) (-21.8391, 58.6184) (-21.9096, 58.6506) (-21.9772, 58.688) (-22.0359, 58.7206) (-22.0924, 58.7571) (-22.1462, 58.7972) (-22.188, 58.8283) (-22.2282, 58.8617) (-22.2666, 58.897) (-22.3049, 58.9323) (-22.3413, 58.9696) (-22.3758, 59.0087) (-22.4079, 59.0452) (-22.4382, 59.0832) (-22.4666, 59.1226) (-22.493, 59.1592) (-22.5178, 59.1971) (-22.5408, 59.2359) (-22.5657, 59.278) (-22.5886, 59.3213) (-22.6092, 59.3656) (-22.6329, 59.4162) (-22.6537, 59.4682) (-22.6715, 59.5212) (-22.6907, 59.578) (-22.7064, 59.636) (-22.7186, 59.6948) (-22.7287, 59.7432) (-22.7363, 59.7921) (-22.7416, 59.8412) (-22.7457, 59.88) (-22.7483, 59.9189) (-22.7494, 59.9579) (-22.7498, 59.9719) (-22.75, 59.986) (-22.75, 60) (-22.75, 60.0174) (-22.7497, 60.0348) (-22.7491, 60.0521) (-22.748, 60.0835) (-22.7459, 60.1149) (-22.7429, 60.1461) (-22.7385, 60.1907) (-22.7321, 60.2351) (-22.7238, 60.2791) (-22.7135, 60.3334) (-22.7003, 60.3871) (-22.6841, 60.4399) (-22.6648, 60.5026) (-22.6414, 60.5641) (-22.6141, 60.6238) (-22.591, 60.6745) (-22.565, 60.7238) (-22.5363, 60.7716) (-22.5113, 60.8134) (-22.4842, 60.8539) (-22.4552, 60.893) (-22.4283, 60.9293) (-22.3998, 60.9643) (-22.3698, 60.998) (-22.3375, 61.0343) (-22.3034, 61.0689) (-22.2678, 61.1019) (-22.227, 61.1395) (-22.1843, 61.1748) (-22.1396, 61.2077) (-22.0923, 61.2426) (-22.0428, 61.2747) (-21.9916, 61.3038) (-21.9405, 61.3329) (-21.8877, 61.359) (-21.8335, 61.3818) (-21.7826, 61.4034) (-21.7304, 61.4221) (-21.6774, 61.4378) (-21.631, 61.4516) (-21.584, 61.4631) (-21.5365, 61.4724) (-21.4925, 61.4809) (-21.4481, 61.4875) (-21.4034, 61.4921) (-21.3622, 61.4964) (-21.3209, 61.4989) (-21.2795, 61.4997) (-21.2696, 61.4999) (-21.2598, 61.5) (-21.25, 61.5) (-21.2184, 61.5) (-21.1869, 61.499) (-21.1554, 61.497) (-21.1107, 61.4942) (-21.0661, 61.4894) (-21.0218, 61.4825) (-20.9741, 61.4752) (-20.9268, 61.4656) (-20.8801, 61.4537) (-20.8266, 61.4401) (-20.774, 61.4235) (-20.7224, 61.4042) (-20.6676, 61.3836) (-20.6141, 61.3598) (-20.5621, 61.333) (-20.5101, 61.3061) (-20.4596, 61.2762) (-20.411, 61.2434) (-20.3652, 61.2125) (-20.3211, 61.1791) (-20.279, 61.1433) (-20.2262, 61.0985) (-20.1765, 61.0499) (-20.1303, 60.9982) (-20.0771, 60.9384) (-20.0286, 60.8744) (-19.9855, 60.8069) (-19.9443, 60.7423) (-19.908, 60.6745) (-19.8771, 60.6042) (-19.8546, 60.5531) (-19.8349, 60.5007) (-19.8182, 60.4473) (-19.8042, 60.4024) (-19.7923, 60.3568) (-19.7826, 60.3108) (-19.7735, 60.2682) (-19.7664, 60.2251) (-19.7611, 60.1819) (-19.7562, 60.1421) (-19.7529, 60.1021) (-19.7513, 60.062) (-19.7504, 60.0413) (-19.75, 60.0207) (-19.75, 60) (-19.75, 59.9892) (-19.7501, 59.9785) (-19.7503, 59.9677) (-19.751, 59.9363) (-19.7527, 59.9049) (-19.7553, 59.8736) (-19.759, 59.8301) (-19.7646, 59.7868) (-19.7721, 59.7437) (-19.7813, 59.6904) (-19.7934, 59.6375) (-19.8084, 59.5855) (-19.8262, 59.5235) (-19.8481, 59.4626) (-19.8738, 59.4034) (-19.8959, 59.3522) (-19.9209, 59.3023) (-19.9487, 59.254) (-19.9729, 59.2117) (-19.9992, 59.1707) (-20.0274, 59.131) (-20.0535, 59.0942) (-20.0813, 59.0586) (-20.1107, 59.0243) (-20.1423, 58.9874) (-20.1757, 58.9521) (-20.2107, 58.9184) (-20.2507, 58.88) (-20.2928, 58.8438) (-20.3367, 58.8101) (-20.3834, 58.7742) (-20.4322, 58.7411) (-20.4828, 58.711) (-20.5343, 58.6804) (-20.5876, 58.6529) (-20.6424, 58.6286) (-20.6949, 58.6053) (-20.7489, 58.585) (-20.8038, 58.5679) (-20.8541, 58.5522) (-20.9053, 58.5392) (-20.957, 58.5289) (-21.0064, 58.5191) (-21.0563, 58.5117) (-21.1064, 58.5069) (-21.1541, 58.5023) (-21.202, 58.5) (-21.25, 58.5) knots 0 0 0 0 0.014027 0.014027 0.014027 0.032151 0.032151 0.032151 0.055886 0.055886 0.055886 0.080494 0.080494 0.080494 0.10188 0.10188 0.10188 0.118509 0.118509 0.118509 0.135113 0.135113 0.135113 0.150598 0.150598 0.150598 0.164992 0.164992 0.164992 0.180561 0.180561 0.180561 0.198348 0.198348 0.198348 0.217433 0.217433 0.217433 0.23315 0.23315 0.23315 0.245536 0.245536 0.245536 0.249999 0.249999 0.249999 0.255524 0.255524 0.255524 0.265505 0.265505 0.265505 0.27974 0.27974 0.27974 0.297306 0.297306 0.297306 0.318194 0.318194 0.318194 0.335939 0.335939 0.335939 0.351456 0.351456 0.351456 0.36584 0.36584 0.36584 0.381321 0.381321 0.381321 0.398988 0.398988 0.398988 0.417741 0.417741 0.417741 0.436466 0.436466 0.436466 0.454074 0.454074 0.454074 0.469453 0.469453 0.469453 0.483718 0.483718 0.483718 0.496876 0.496876 0.496876 0.499998 0.499998 0.499998 0.51003 0.51003 0.51003 0.524271 0.524271 0.524271 0.539608 0.539608 0.539608 0.557137 0.557137 0.557137 0.575761 0.575761 0.575761 0.594424 0.594424 0.594424 0.612031 0.612031 0.612031 0.634137 0.634137 0.634137 0.659646 0.659646 0.659646 0.684077 0.684077 0.684077 0.701865 0.701865 0.701865 0.716826 0.716826 0.716826 0.730685 0.730685 0.730685 0.743429 0.743429 0.743429 0.749997 0.749997 0.749997 0.753416 0.753416 0.753416 0.763398 0.763398 0.763398 0.777282 0.777282 0.777282 0.794497 0.794497 0.794497 0.815037 0.815037 0.815037 0.832783 0.832783 0.832783 0.848301 0.848301 0.848301 0.862688 0.862688 0.862688 0.878174 0.878174 0.878174 0.895845 0.895845 0.895845 0.914604 0.914604 0.914604 0.933679 0.933679 0.933679 0.951984 0.951984 0.951984 0.968755 0.968755 0.968755 0.984759 0.984759 0.984759 1 1 1 1 projected
  spline S5 degree 3 poles (-21.25, 38.5) (-21.2941, 38.5) (-21.3383, 38.5019) (-21.3822, 38.5058) (-21.439, 38.5109) (-21.4955, 38.5191) (-21.5514, 38.5306) (-21.6245, 38.5456) (-21.6965, 38.566) (-21.7665, 38.5917) (-21.8391, 38.6184) (-21.9096, 38.6506) (-21.9772, 38.688) (-22.0359, 38.7206) (-22.0924, 38.7571) (-22.1462, 38.7972) (-22.188, 38.8283) (-22.2282, 38.8617) (-22.2666, 38.897) (-22.3049, 38.9323) (-22.3413, 38.9696) (-22.3758, 39.0087) (-22.4079, 39.0452) (-22.4382, 39.0832) (-22.4666, 39.1226) (-22.493, 39.1592) (-22.5178, 39.1971) (-22.5408, 39.2359) (-22.5657, 39.278) (-22.5886, 39.3213) (-22.6092, 39.3656) (-22.6329, 39.4162) (-22.6537, 39.4682) (-22.6715, 39.5212) (-22.6907, 39.578) (-22.7064, 39.636) (-22.7186, 39.6948) (-22.7287, 39.7432) (-22.7363, 39.7921) (-22.7416, 39.8412) (-22.7457, 39.88) (-22.7483, 39.9189) (-22.7494, 39.9579) (-22.7498, 39.9719) (-22.75, 39.986) (-22.75, 40) (-22.75, 40.0174) (-22.7497, 40.0348) (-22.7491, 40.0521) (-22.748, 40.0835) (-22.7459, 40.1149) (-22.7429, 40.1461) (-22.7385, 40.1907) (-22.7321, 40.2351) (-22.7238, 40.2791) (-22.7135, 40.3334) (-22.7003, 40.3871) (-22.6841, 40.4399) (-22.6648, 40.5026) (-22.6414, 40.5641) (-22.6141, 40.6238) (-22.591, 40.6745) (-22.565, 40.7238) (-22.5363, 40.7716) (-22.5113, 40.8134) (-22.4842, 40.8539) (-22.4552, 40.893) (-22.4283, 40.9293) (-22.3998, 40.9643) (-22.3698, 40.998) (-22.3375, 41.0343) (-22.3034, 41.0689) (-22.2678, 41.1019) (-22.227, 41.1395) (-22.1843, 41.1748) (-22.1396, 41.2077) (-22.0923, 41.2426) (-22.0428, 41.2747) (-21.9916, 41.3038) (-21.9405, 41.3329) (-21.8877, 41.359) (-21.8335, 41.3818) (-21.7826, 41.4034) (-21.7304, 41.4221) (-21.6774, 41.4378) (-21.631, 41.4516) (-21.584, 41.4631) (-21.5365, 41.4724) (-21.4925, 41.4809) (-21.4481, 41.4875) (-21.4034, 41.4921) (-21.3622, 41.4964) (-21.3209, 41.4989) (-21.2795, 41.4997) (-21.2696, 41.4999) (-21.2598, 41.5) (-21.25, 41.5) (-21.2184, 41.5) (-21.1869, 41.499) (-21.1554, 41.497) (-21.1107, 41.4942) (-21.0661, 41.4894) (-21.0218, 41.4825) (-20.9741, 41.4752) (-20.9268, 41.4656) (-20.8801, 41.4537) (-20.8266, 41.4401) (-20.774, 41.4235) (-20.7224, 41.4042) (-20.6676, 41.3836) (-20.6141, 41.3598) (-20.5621, 41.333) (-20.5101, 41.3061) (-20.4596, 41.2762) (-20.411, 41.2434) (-20.3652, 41.2125) (-20.3211, 41.1791) (-20.279, 41.1433) (-20.2262, 41.0985) (-20.1765, 41.0499) (-20.1303, 40.9982) (-20.0771, 40.9384) (-20.0286, 40.8744) (-19.9855, 40.8069) (-19.9443, 40.7423) (-19.908, 40.6745) (-19.8771, 40.6042) (-19.8546, 40.5531) (-19.8349, 40.5007) (-19.8182, 40.4473) (-19.8042, 40.4024) (-19.7923, 40.3568) (-19.7826, 40.3108) (-19.7735, 40.2682) (-19.7664, 40.2251) (-19.7611, 40.1819) (-19.7562, 40.1421) (-19.7529, 40.1021) (-19.7513, 40.062) (-19.7504, 40.0413) (-19.75, 40.0207) (-19.75, 40) (-19.75, 39.9892) (-19.7501, 39.9785) (-19.7503, 39.9677) (-19.751, 39.9363) (-19.7527, 39.9049) (-19.7553, 39.8736) (-19.759, 39.8301) (-19.7646, 39.7868) (-19.7721, 39.7437) (-19.7813, 39.6904) (-19.7934, 39.6375) (-19.8084, 39.5855) (-19.8262, 39.5235) (-19.8481, 39.4626) (-19.8738, 39.4034) (-19.8959, 39.3522) (-19.9209, 39.3023) (-19.9487, 39.254) (-19.9729, 39.2117) (-19.9992, 39.1707) (-20.0274, 39.131) (-20.0535, 39.0942) (-20.0813, 39.0586) (-20.1107, 39.0243) (-20.1423, 38.9874) (-20.1757, 38.9521) (-20.2107, 38.9184) (-20.2507, 38.88) (-20.2928, 38.8438) (-20.3367, 38.8101) (-20.3834, 38.7742) (-20.4322, 38.7411) (-20.4828, 38.711) (-20.5343, 38.6804) (-20.5876, 38.6529) (-20.6424, 38.6286) (-20.6949, 38.6053) (-20.7489, 38.585) (-20.8038, 38.5679) (-20.8541, 38.5522) (-20.9053, 38.5392) (-20.957, 38.5289) (-21.0064, 38.5191) (-21.0563, 38.5117) (-21.1064, 38.5069) (-21.1541, 38.5023) (-21.202, 38.5) (-21.25, 38.5) knots 0 0 0 0 0.014027 0.014027 0.014027 0.032151 0.032151 0.032151 0.055886 0.055886 0.055886 0.080494 0.080494 0.080494 0.10188 0.10188 0.10188 0.118509 0.118509 0.118509 0.135113 0.135113 0.135113 0.150598 0.150598 0.150598 0.164992 0.164992 0.164992 0.180561 0.180561 0.180561 0.198348 0.198348 0.198348 0.217433 0.217433 0.217433 0.23315 0.23315 0.23315 0.245536 0.245536 0.245536 0.249999 0.249999 0.249999 0.255524 0.255524 0.255524 0.265505 0.265505 0.265505 0.27974 0.27974 0.27974 0.297306 0.297306 0.297306 0.318194 0.318194 0.318194 0.335939 0.335939 0.335939 0.351456 0.351456 0.351456 0.36584 0.36584 0.36584 0.381321 0.381321 0.381321 0.398988 0.398988 0.398988 0.417741 0.417741 0.417741 0.436466 0.436466 0.436466 0.454074 0.454074 0.454074 0.469453 0.469453 0.469453 0.483718 0.483718 0.483718 0.496876 0.496876 0.496876 0.499998 0.499998 0.499998 0.51003 0.51003 0.51003 0.524271 0.524271 0.524271 0.539608 0.539608 0.539608 0.557137 0.557137 0.557137 0.575761 0.575761 0.575761 0.594424 0.594424 0.594424 0.612031 0.612031 0.612031 0.634137 0.634137 0.634137 0.659646 0.659646 0.659646 0.684077 0.684077 0.684077 0.701865 0.701865 0.701865 0.716826 0.716826 0.716826 0.730685 0.730685 0.730685 0.743429 0.743429 0.743429 0.749997 0.749997 0.749997 0.753416 0.753416 0.753416 0.763398 0.763398 0.763398 0.777282 0.777282 0.777282 0.794497 0.794497 0.794497 0.815037 0.815037 0.815037 0.832783 0.832783 0.832783 0.848301 0.848301 0.848301 0.862688 0.862688 0.862688 0.878174 0.878174 0.878174 0.895845 0.895845 0.895845 0.914604 0.914604 0.914604 0.933679 0.933679 0.933679 0.951984 0.951984 0.951984 0.968755 0.968755 0.968755 0.984759 0.984759 0.984759 1 1 1 1 projected
  spline S6 degree 3 poles (-21.25, 18.5) (-21.2941, 18.5) (-21.3383, 18.5019) (-21.3822, 18.5058) (-21.439, 18.5109) (-21.4955, 18.5191) (-21.5514, 18.5306) (-21.6245, 18.5456) (-21.6965, 18.566) (-21.7665, 18.5917) (-21.8391, 18.6184) (-21.9096, 18.6506) (-21.9772, 18.688) (-22.0359, 18.7206) (-22.0924, 18.7571) (-22.1462, 18.7972) (-22.188, 18.8283) (-22.2282, 18.8617) (-22.2666, 18.897) (-22.3049, 18.9323) (-22.3413, 18.9696) (-22.3758, 19.0087) (-22.4079, 19.0452) (-22.4382, 19.0832) (-22.4666, 19.1226) (-22.493, 19.1592) (-22.5178, 19.1971) (-22.5408, 19.2359) (-22.5657, 19.278) (-22.5886, 19.3213) (-22.6092, 19.3656) (-22.6329, 19.4162) (-22.6537, 19.4682) (-22.6715, 19.5212) (-22.6907, 19.578) (-22.7064, 19.636) (-22.7186, 19.6948) (-22.7287, 19.7432) (-22.7363, 19.7921) (-22.7416, 19.8412) (-22.7457, 19.88) (-22.7483, 19.9189) (-22.7494, 19.9579) (-22.7498, 19.9719) (-22.75, 19.986) (-22.75, 20) (-22.75, 20.0174) (-22.7497, 20.0348) (-22.7491, 20.0521) (-22.748, 20.0835) (-22.7459, 20.1149) (-22.7429, 20.1461) (-22.7385, 20.1907) (-22.7321, 20.2351) (-22.7238, 20.2791) (-22.7135, 20.3334) (-22.7003, 20.3871) (-22.6841, 20.4399) (-22.6648, 20.5026) (-22.6414, 20.5641) (-22.6141, 20.6238) (-22.591, 20.6745) (-22.565, 20.7238) (-22.5363, 20.7716) (-22.5113, 20.8134) (-22.4842, 20.8539) (-22.4552, 20.893) (-22.4283, 20.9293) (-22.3998, 20.9643) (-22.3698, 20.998) (-22.3375, 21.0343) (-22.3034, 21.0689) (-22.2678, 21.1019) (-22.227, 21.1395) (-22.1843, 21.1748) (-22.1396, 21.2077) (-22.0923, 21.2426) (-22.0428, 21.2747) (-21.9916, 21.3038) (-21.9405, 21.3329) (-21.8877, 21.359) (-21.8335, 21.3818) (-21.7826, 21.4034) (-21.7304, 21.4221) (-21.6774, 21.4378) (-21.631, 21.4516) (-21.584, 21.4631) (-21.5365, 21.4724) (-21.4925, 21.4809) (-21.4481, 21.4875) (-21.4034, 21.4921) (-21.3622, 21.4964) (-21.3209, 21.4989) (-21.2795, 21.4997) (-21.2696, 21.4999) (-21.2598, 21.5) (-21.25, 21.5) (-21.2184, 21.5) (-21.1869, 21.499) (-21.1554, 21.497) (-21.1107, 21.4942) (-21.0661, 21.4894) (-21.0218, 21.4825) (-20.9741, 21.4752) (-20.9268, 21.4656) (-20.8801, 21.4537) (-20.8266, 21.4401) (-20.774, 21.4235) (-20.7224, 21.4042) (-20.6676, 21.3836) (-20.6141, 21.3598) (-20.5621, 21.333) (-20.5101, 21.3061) (-20.4596, 21.2762) (-20.411, 21.2434) (-20.3652, 21.2125) (-20.3211, 21.1791) (-20.279, 21.1433) (-20.2262, 21.0985) (-20.1765, 21.0499) (-20.1303, 20.9982) (-20.0771, 20.9384) (-20.0286, 20.8744) (-19.9855, 20.8069) (-19.9443, 20.7423) (-19.908, 20.6745) (-19.8771, 20.6042) (-19.8546, 20.5531) (-19.8349, 20.5007) (-19.8182, 20.4473) (-19.8042, 20.4024) (-19.7923, 20.3568) (-19.7826, 20.3108) (-19.7735, 20.2682) (-19.7664, 20.2251) (-19.7611, 20.1819) (-19.7562, 20.1421) (-19.7529, 20.1021) (-19.7513, 20.062) (-19.7504, 20.0413) (-19.75, 20.0207) (-19.75, 20) (-19.75, 19.9892) (-19.7501, 19.9785) (-19.7503, 19.9677) (-19.751, 19.9363) (-19.7527, 19.9049) (-19.7553, 19.8736) (-19.759, 19.8301) (-19.7646, 19.7868) (-19.7721, 19.7437) (-19.7813, 19.6904) (-19.7934, 19.6375) (-19.8084, 19.5855) (-19.8262, 19.5235) (-19.8481, 19.4626) (-19.8738, 19.4034) (-19.8959, 19.3522) (-19.9209, 19.3023) (-19.9487, 19.254) (-19.9729, 19.2117) (-19.9992, 19.1707) (-20.0274, 19.131) (-20.0535, 19.0942) (-20.0813, 19.0586) (-20.1107, 19.0243) (-20.1423, 18.9874) (-20.1757, 18.9521) (-20.2107, 18.9184) (-20.2507, 18.88) (-20.2928, 18.8438) (-20.3367, 18.8101) (-20.3834, 18.7742) (-20.4322, 18.7411) (-20.4828, 18.711) (-20.5343, 18.6804) (-20.5876, 18.6529) (-20.6424, 18.6286) (-20.6949, 18.6053) (-20.7489, 18.585) (-20.8038, 18.5679) (-20.8541, 18.5522) (-20.9053, 18.5392) (-20.957, 18.5289) (-21.0064, 18.5191) (-21.0563, 18.5117) (-21.1064, 18.5069) (-21.1541, 18.5023) (-21.202, 18.5) (-21.25, 18.5) knots 0 0 0 0 0.014027 0.014027 0.014027 0.032151 0.032151 0.032151 0.055886 0.055886 0.055886 0.080494 0.080494 0.080494 0.10188 0.10188 0.10188 0.118509 0.118509 0.118509 0.135113 0.135113 0.135113 0.150598 0.150598 0.150598 0.164992 0.164992 0.164992 0.180561 0.180561 0.180561 0.198348 0.198348 0.198348 0.217433 0.217433 0.217433 0.23315 0.23315 0.23315 0.245536 0.245536 0.245536 0.249999 0.249999 0.249999 0.255524 0.255524 0.255524 0.265505 0.265505 0.265505 0.27974 0.27974 0.27974 0.297306 0.297306 0.297306 0.318194 0.318194 0.318194 0.335939 0.335939 0.335939 0.351456 0.351456 0.351456 0.36584 0.36584 0.36584 0.381321 0.381321 0.381321 0.398988 0.398988 0.398988 0.417741 0.417741 0.417741 0.436466 0.436466 0.436466 0.454074 0.454074 0.454074 0.469453 0.469453 0.469453 0.483718 0.483718 0.483718 0.496876 0.496876 0.496876 0.499998 0.499998 0.499998 0.51003 0.51003 0.51003 0.524271 0.524271 0.524271 0.539608 0.539608 0.539608 0.557137 0.557137 0.557137 0.575761 0.575761 0.575761 0.594424 0.594424 0.594424 0.612031 0.612031 0.612031 0.634137 0.634137 0.634137 0.659646 0.659646 0.659646 0.684077 0.684077 0.684077 0.701865 0.701865 0.701865 0.716826 0.716826 0.716826 0.730685 0.730685 0.730685 0.743429 0.743429 0.743429 0.749997 0.749997 0.749997 0.753416 0.753416 0.753416 0.763398 0.763398 0.763398 0.777282 0.777282 0.777282 0.794497 0.794497 0.794497 0.815037 0.815037 0.815037 0.832783 0.832783 0.832783 0.848301 0.848301 0.848301 0.862688 0.862688 0.862688 0.878174 0.878174 0.878174 0.895845 0.895845 0.895845 0.914604 0.914604 0.914604 0.933679 0.933679 0.933679 0.951984 0.951984 0.951984 0.968755 0.968755 0.968755 0.984759 0.984759 0.984759 1 1 1 1 projected
  spline S7 degree 3 poles (-21.25, 78.5) (-21.2941, 78.5) (-21.3383, 78.5019) (-21.3822, 78.5058) (-21.439, 78.5109) (-21.4955, 78.5191) (-21.5514, 78.5306) (-21.6245, 78.5456) (-21.6965, 78.566) (-21.7665, 78.5917) (-21.8391, 78.6184) (-21.9096, 78.6506) (-21.9772, 78.688) (-22.0359, 78.7206) (-22.0924, 78.7571) (-22.1462, 78.7972) (-22.188, 78.8283) (-22.2282, 78.8617) (-22.2666, 78.897) (-22.3049, 78.9323) (-22.3413, 78.9696) (-22.3758, 79.0087) (-22.4079, 79.0452) (-22.4382, 79.0832) (-22.4666, 79.1226) (-22.493, 79.1592) (-22.5178, 79.1971) (-22.5408, 79.2359) (-22.5657, 79.278) (-22.5886, 79.3213) (-22.6092, 79.3656) (-22.6329, 79.4162) (-22.6537, 79.4682) (-22.6715, 79.5212) (-22.6907, 79.578) (-22.7064, 79.636) (-22.7186, 79.6948) (-22.7287, 79.7432) (-22.7363, 79.7921) (-22.7416, 79.8412) (-22.7457, 79.88) (-22.7483, 79.9189) (-22.7494, 79.9579) (-22.7498, 79.9719) (-22.75, 79.986) (-22.75, 80) (-22.75, 80.0174) (-22.7497, 80.0348) (-22.7491, 80.0521) (-22.748, 80.0835) (-22.7459, 80.1149) (-22.7429, 80.1461) (-22.7385, 80.1907) (-22.7321, 80.2351) (-22.7238, 80.2791) (-22.7135, 80.3334) (-22.7003, 80.3871) (-22.6841, 80.4399) (-22.6648, 80.5026) (-22.6414, 80.5641) (-22.6141, 80.6238) (-22.591, 80.6745) (-22.565, 80.7238) (-22.5363, 80.7716) (-22.5113, 80.8134) (-22.4842, 80.8539) (-22.4552, 80.893) (-22.4283, 80.9293) (-22.3998, 80.9643) (-22.3698, 80.998) (-22.3375, 81.0343) (-22.3034, 81.0689) (-22.2678, 81.1019) (-22.227, 81.1395) (-22.1843, 81.1748) (-22.1396, 81.2077) (-22.0923, 81.2426) (-22.0428, 81.2747) (-21.9916, 81.3038) (-21.9405, 81.3329) (-21.8877, 81.359) (-21.8335, 81.3818) (-21.7826, 81.4034) (-21.7304, 81.4221) (-21.6774, 81.4378) (-21.631, 81.4516) (-21.584, 81.4631) (-21.5365, 81.4724) (-21.4925, 81.4809) (-21.4481, 81.4875) (-21.4034, 81.4921) (-21.3622, 81.4964) (-21.3209, 81.4989) (-21.2795, 81.4997) (-21.2696, 81.4999) (-21.2598, 81.5) (-21.25, 81.5) (-21.2184, 81.5) (-21.1869, 81.499) (-21.1554, 81.497) (-21.1107, 81.4942) (-21.0661, 81.4894) (-21.0218, 81.4825) (-20.9741, 81.4752) (-20.9268, 81.4656) (-20.8801, 81.4537) (-20.8266, 81.4401) (-20.774, 81.4235) (-20.7224, 81.4042) (-20.6676, 81.3836) (-20.6141, 81.3598) (-20.5621, 81.333) (-20.5101, 81.3061) (-20.4596, 81.2762) (-20.411, 81.2434) (-20.3652, 81.2125) (-20.3211, 81.1791) (-20.279, 81.1433) (-20.2262, 81.0985) (-20.1765, 81.0499) (-20.1303, 80.9982) (-20.0771, 80.9384) (-20.0286, 80.8744) (-19.9855, 80.8069) (-19.9443, 80.7423) (-19.908, 80.6745) (-19.8771, 80.6042) (-19.8546, 80.5531) (-19.8349, 80.5007) (-19.8182, 80.4473) (-19.8042, 80.4024) (-19.7923, 80.3568) (-19.7826, 80.3108) (-19.7735, 80.2682) (-19.7664, 80.2251) (-19.7611, 80.1819) (-19.7562, 80.1421) (-19.7529, 80.1021) (-19.7513, 80.062) (-19.7504, 80.0413) (-19.75, 80.0207) (-19.75, 80) (-19.75, 79.9892) (-19.7501, 79.9785) (-19.7503, 79.9677) (-19.751, 79.9363) (-19.7527, 79.9049) (-19.7553, 79.8736) (-19.759, 79.8301) (-19.7646, 79.7868) (-19.7721, 79.7437) (-19.7813, 79.6904) (-19.7934, 79.6375) (-19.8084, 79.5855) (-19.8262, 79.5235) (-19.8481, 79.4626) (-19.8738, 79.4034) (-19.8959, 79.3522) (-19.9209, 79.3023) (-19.9487, 79.254) (-19.9729, 79.2117) (-19.9992, 79.1707) (-20.0274, 79.131) (-20.0535, 79.0942) (-20.0813, 79.0586) (-20.1107, 79.0243) (-20.1423, 78.9874) (-20.1757, 78.9521) (-20.2107, 78.9184) (-20.2507, 78.88) (-20.2928, 78.8438) (-20.3367, 78.8101) (-20.3834, 78.7742) (-20.4322, 78.7411) (-20.4828, 78.711) (-20.5343, 78.6804) (-20.5876, 78.6529) (-20.6424, 78.6286) (-20.6949, 78.6053) (-20.7489, 78.585) (-20.8038, 78.5679) (-20.8541, 78.5522) (-20.9053, 78.5392) (-20.957, 78.5289) (-21.0064, 78.5191) (-21.0563, 78.5117) (-21.1064, 78.5069) (-21.1541, 78.5023) (-21.202, 78.5) (-21.25, 78.5) knots 0 0 0 0 0.014027 0.014027 0.014027 0.032151 0.032151 0.032151 0.055886 0.055886 0.055886 0.080494 0.080494 0.080494 0.10188 0.10188 0.10188 0.118509 0.118509 0.118509 0.135113 0.135113 0.135113 0.150598 0.150598 0.150598 0.164992 0.164992 0.164992 0.180561 0.180561 0.180561 0.198348 0.198348 0.198348 0.217433 0.217433 0.217433 0.23315 0.23315 0.23315 0.245536 0.245536 0.245536 0.249999 0.249999 0.249999 0.255524 0.255524 0.255524 0.265505 0.265505 0.265505 0.27974 0.27974 0.27974 0.297306 0.297306 0.297306 0.318194 0.318194 0.318194 0.335939 0.335939 0.335939 0.351456 0.351456 0.351456 0.36584 0.36584 0.36584 0.381321 0.381321 0.381321 0.398988 0.398988 0.398988 0.417741 0.417741 0.417741 0.436466 0.436466 0.436466 0.454074 0.454074 0.454074 0.469453 0.469453 0.469453 0.483718 0.483718 0.483718 0.496876 0.496876 0.496876 0.499998 0.499998 0.499998 0.51003 0.51003 0.51003 0.524271 0.524271 0.524271 0.539608 0.539608 0.539608 0.557137 0.557137 0.557137 0.575761 0.575761 0.575761 0.594424 0.594424 0.594424 0.612031 0.612031 0.612031 0.634137 0.634137 0.634137 0.659646 0.659646 0.659646 0.684077 0.684077 0.684077 0.701865 0.701865 0.701865 0.716826 0.716826 0.716826 0.730685 0.730685 0.730685 0.743429 0.743429 0.743429 0.749997 0.749997 0.749997 0.753416 0.753416 0.753416 0.763398 0.763398 0.763398 0.777282 0.777282 0.777282 0.794497 0.794497 0.794497 0.815037 0.815037 0.815037 0.832783 0.832783 0.832783 0.848301 0.848301 0.848301 0.862688 0.862688 0.862688 0.878174 0.878174 0.878174 0.895845 0.895845 0.895845 0.914604 0.914604 0.914604 0.933679 0.933679 0.933679 0.951984 0.951984 0.951984 0.968755 0.968755 0.968755 0.984759 0.984759 0.984759 1 1 1 1 projected
  point P0 (0, 0)
  point P1 (-76.75, 18.5)
  point P2 (-76.75, 38.5)
  point P3 (-76.75, 58.5)
  point P4 (-76.75, 78.5)
  point P5 (-21.25, 58.5)
  point P6 (-21.25, 38.5)
  point P7 (-21.25, 18.5)
  point P8 (-21.25, 78.5)
extrude "Выдавливание6" cut sketch "Эскиз7" against normal blind 10
